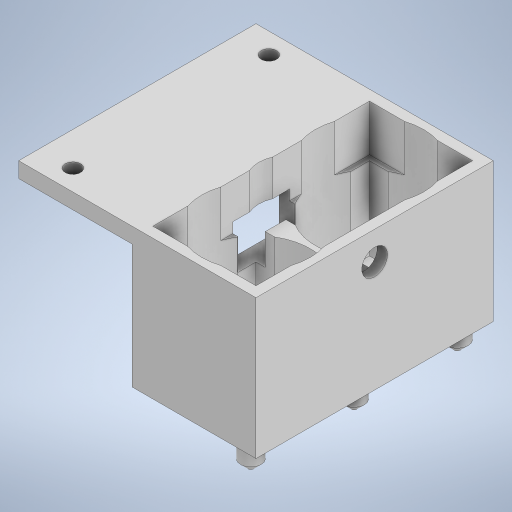
# Autodesk Inventor part: Suporte Eletroimã
Saved by Autodesk Inventor 2023 (Build 270158000, 158)
## iProperties
Created: 2023-03-07
Part Number: Suporte Eletroimã
Material: Genérico
Document SubType Name: Modeling
Designer: Inteli
Density: 1 g/cm^3
Appearance: Padrão
Author: Inteli
Autodesk Inventor part; units mm, degrees
ref_plane "YZ Plane" through (0, 0, 0) normal (1, 0, 0) x (0, 1, 0)
ref_plane "XZ Plane" through (0, 0, 0) normal (0, 1, 0) x (-1, 0, 0)
ref_plane "XY Plane" through (0, 0, 0) normal (0, 0, 1) x (1, 0, 0)
sketch "Esboço1" plane through (0, 0, 0) normal (0, 1, 0) x (-1, 0, 0)
  circle A0 centre (0, 11) radius 10.5
  circle A1 centre (0, -11) radius 10.5
  line L0 (9, 2) -> (-9, 2)
  line L1 (-9, -2) -> (9, -2)
  line L2 (9, 20) -> (-9, 20)
  line L3 (-9, -20) -> (9, -20)
  line L4 (12, 23) -> (-12, 23)
  line L5 (-12, 23) -> (-12, -23)
  line L6 (-12, -23) -> (12, -23)
  line L7 (12, -23) -> (12, 23)
  line L8 (9, -20) -> (9, -2)
  line L9 (9, 2) -> (9, 20)
  line L10 (-9, 20) -> (-9, 2)
  line L11 (-9, -2) -> (-9, -20)
  point P0 (-9, 5.5917)
  point P1 (-9, 16.4083)
  point P2 (-5.4083, 20)
  point P3 (5.4083, 20)
  point P4 (9, 16.4083)
  point P5 (9, 5.5917)
  point P6 (5.4083, 2)
  point P7 (-5.4083, 2)
  point P8 (-9, -5.5917)
  point P9 (-5.4083, -2)
  point P10 (5.4083, -2)
  point P11 (9, -5.5917)
  point P12 (9, -16.4083)
  point P13 (5.4083, -20)
  point P14 (-5.4083, -20)
  point P15 (-9, -16.4083)
  point P16 (0, 0)
  point P17 (0, 21.5)
  point P18 (0, 21.5)
  dimension "d94" = 21
  dimension "d16" = 40
  dimension "d17" = 18
  dimension "d18" = 24
  dimension "d61" = 46
  dimension "d62" = 22
  dimension "d93" = 21
  constraints: 24 end point, 8 parallel, 3 horizontal, 3 perpendicular, 2 coincident, 1 centre point, 3 other
  measures "d16" distance of L3.start L2.end
  measures "d17" distance of L3.start L3.end
  measures "d18" distance of L6.end L5.end
  measures "d61" distance of L4.end L5.end
  measures "d62" distance of point (0, 11) A1.centre
  measures "d93" diameter of A1
extrude "Base Principal dos Imãs" add sketch "Esboço1" along normal blind 25
sketch "Esboço9" plane through (0, 0, 0) normal (0, -1, 0) x (1, 0, 0)
  line L0 (-12, 23) -> (12, 23) projected
  line L1 (12, -23) -> (-12, -23) projected
  line L2 (12, 23) -> (-12, 23)
  line L3 (-12, 23) -> (-12, -23)
  line L4 (-12, -23) -> (12, -23)
  line L5 (12, -23) -> (12, 23)
  point P0 (0, 0)
  point P1 (12, -23)
  constraints: 8 end point, 2 parallel, 1 horizontal, 1 perpendicular
extrude "Fundo" add sketch "Esboço9" along normal blind 2
sketch "Esboço13" plane through (0, 25, 0) normal (0, 1, 0) x (1, 0, 0)
  line L0 (10, 21) -> (-10, 21)
  line L1 (-10, 21) -> (-10, -21)
  line L2 (-10, -21) -> (10, -21)
  line L3 (10, -21) -> (10, 21)
  line L4 (10, 21) -> (-10, -21) construction
  line L5 (-10, 21) -> (10, -21) construction
  point P0 (0, 0)
  dimension "d84" = 20
  dimension "d85" = 42
  constraints: 12 end point, 2 midpoint, 2 parallel, 1 horizontal, 1 perpendicular
  measures "d84" distance of L2.end L1.end
  measures "d85" distance of L1.end L0.end
extrude "PCB / Tampa" cut sketch "Esboço13" against normal blind 9
sketch "Esboço14" plane through (0, 25, 0) normal (0, 1, 0) x (1, 0, 0)
  line L0 (-9, -2) -> (-5.4083, -2) projected
  line L1 (-7.2042, -2) -> (-9, -3.7958)
  line L2 (-9, -5.5917) -> (-9, -2) projected
  line L3 (-7.2042, -2) -> (-7.2042, 2)
  line L4 (-9, 2) -> (-5.4083, 2) projected
  line L5 (-9, 2) -> (-9, 5.5917) projected
  line L6 (-9, 3.7958) -> (-7.2042, 2)
  arc A0 (-9, 3.7958) -> (-9, -3.7958) centre (-4.7924, 0) ccw
  point P0 (0, 0)
  constraints: 6 end point, 4 midpoint, 2 point on circle, 1 centre point, 1 perpendicular
extrude "Espaço Fio (Validar)" cut sketch "Esboço14" against normal blind 15
sketch "Esboço15" plane through (10, 25, -21) normal (-1, 0, 0) x (0, 0, 1)
  circle A0 centre (21, -5.5) radius 2.5
  point P0 (21, -25)
  dimension "d90" = 5
  constraints: 1 centre point
  measures "d90" diameter of A0
extrude "Furo Led" cut sketch "Esboço15" against normal up to surface (2 mm away)
sketch "Esboço16" plane through (0, -2, 0) normal (0, -1, 0) x (1, 0, 0)
  circle A0 centre (8, 0) radius 2
  line L0 (12, 23) -> (-12, 23) projected
  circle A1 centre (8, 20) radius 2.007
  circle A2 centre (8, -20) radius 2.1182
  line L1 (-12, -23) -> (12, -23) projected
  line L2 (12, -23) -> (12, 23) projected
  point P0 (0, 0)
  dimension "d100" = 4
  dimension "d101" = 3
  dimension "d102" = 4
  dimension "d103" = 4
  dimension "d104" = 4
  dimension "d105" = 3
  constraints: 3 centre point
  measures "d100" diameter of A0
  measures "d101" distance from line of A1.centre L0
  measures "d102" distance from line of L2 A1.centre
  measures "d103" distance from line of A0.centre L2
  measures "d104" distance from line of A2.centre L2
  measures "d105" distance from line of L1 A2.centre
extrude "Rastel" add sketch "Esboço16" along normal blind 5
chamfer "Chanfro1" distance 1.5 angle 45 3 edges at (5.993, -7, 20) (6, -7, 0) (5.8818, -7, -20)
sketch "Esboço17" plane through (-12, 25, -23) normal (-1, 0, 0) x (0, 0, 1)
  line L0 (0, -27) -> (0, 0) projected
  line L1 (46, -27) -> (46, 0) projected
  line L2 (0, 0) -> (46, 0)
  line L3 (46, 0) -> (46, -3)
  line L4 (46, -3) -> (0, -3)
  line L5 (0, -3) -> (0, 0)
  point P0 (23, -25)
  point P1 (0, -3)
  dimension "d109" = 3
  constraints: 8 end point, 2 parallel, 1 horizontal, 1 perpendicular, 1 point on line
  measures "d109" distance of L2.end L3.end
extrude "Suporte IV" add sketch "Esboço17" along normal blind 22
sketch "Esboço18" plane through (-12, 22, -23) normal (0, -1, 0) x (1, 0, 0)
  line L0 (-22, 0) -> (0, 0)
  line L1 (-22, 46) -> (-8, 46)
  line L2 (-22, 46) -> (-22, 0) projected
  line L3 (-22, 0) -> (-22, 46)
  circle A0 centre (-15.5, 4) radius 1.5
  circle A1 centre (-15.5, 42) radius 1.5
  point P0 (12, 23)
  dimension "d115" = 3
  dimension "d116" = 3
  constraints: 6 end point, 2 centre point, 1 vertical
  measures "d115" diameter of A0
  measures "d116" diameter of A1
extrude "Furos Suporte IV" cut sketch "Esboço18" against normal up to surface (3 mm away)
sketch "Esboço19" plane through (-12, -2, -23) normal (-1, 0, 0) x (0, 0, 1)
  line L0 (46, 0) -> (0, 0) projected
  line L1 (17.5, 20) -> (28.5, 20)
  line L2 (28.5, 20) -> (28.5, 12)
  line L3 (28.5, 12) -> (17.5, 12)
  line L4 (17.5, 12) -> (17.5, 20)
  line L5 (0, 24) -> (46, 24) projected
  point P0 (23, 2)
  dimension "d123" = 11
  dimension "d124" = 8
  dimension "d125" = 4
  constraints: 8 end point, 2 parallel, 1 horizontal, 1 perpendicular
  measures "d123" distance of L2.end L3.end
  measures "d124" distance of L1.end L2.end
  measures "d125" distance between parallel lines of L1 L5
extrude "Furo IV" cut sketch "Esboço19" against normal up to surface (3 mm away)
